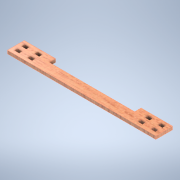
# Autodesk Inventor part: DoorFrameTop
Saved by Autodesk Inventor 2022.2 (Build 262287000, 287)
## iProperties
Created: 2023-03-05
Part Number: DoorFrameTop
Material: Wood (Oak)
Document SubType Name: Modeling
Designer: jaege
Density: 0.76 g/cm^3
Appearance: Red Oak - Natural Low Gloss
Author: jaege
Autodesk Inventor part; units mm, degrees
ref_plane "YZ Plane" through (0, 0, 0) normal (1, 0, 0) x (0, 1, 0)
ref_plane "XZ Plane" through (0, 0, 0) normal (0, 1, 0) x (-1, 0, 0)
ref_plane "XY Plane" through (0, 0, 0) normal (0, 0, 1) x (1, 0, 0)
sketch "Sketch1" plane through (0, 0, 0) normal (0, 1, 0) x (-1, 0, 0)
  line L0 (92, -20.8) -> (53, -20.8)
  line L1 (53, -20.8) -> (53, -12.8)
  line L2 (53, 0) -> (92, 0)
  line L3 (92, 0) -> (92, -20.8)
  line L4 (53, 0) -> (-53, 0)
  line L5 (-53, 0) -> (-53, -12.8) construction
  line L6 (-53, -12.8) -> (53, -12.8)
  line L7 (53, -12.8) -> (53, 0) construction
  line L8 (-53, 0) -> (-92, 0)
  line L9 (-92, 0) -> (-92, -20.8)
  line L10 (-92, -20.8) -> (-53, -20.8)
  line L11 (-53, -20.8) -> (-53, -12.8)
  line L12 (0, -12.8) -> (0, 0)
  line L13 (92, -16.8) -> (-92, -16.8) construction
  line L14 (92, -8) -> (-92, -8) construction
  line L15 (53, -12.8) -> (53, 0) construction
  line L16 (-53, -12.8) -> (-53, 0) construction
  line L17 (92, -4) -> (-92, -4) construction
  line L18 (87.5, -16.8) -> (81.5, -16.8)
  line L19 (81.5, -16.8) -> (81.5, -12.8)
  line L20 (81.5, -12.8) -> (87.5, -12.8)
  line L21 (87.5, -12.8) -> (87.5, -16.8)
  line L22 (71.5, -16.8) -> (65.5, -16.8)
  line L23 (65.5, -16.8) -> (65.5, -12.8)
  line L24 (65.5, -12.8) -> (71.5, -12.8)
  line L25 (71.5, -12.8) -> (71.5, -16.8)
  line L26 (-65.5, -16.8) -> (-71.5, -16.8)
  line L27 (-71.5, -16.8) -> (-71.5, -12.8)
  line L28 (-71.5, -12.8) -> (-65.5, -12.8)
  line L29 (-65.5, -12.8) -> (-65.5, -16.8)
  line L30 (-81.5, -16.8) -> (-87.5, -16.8)
  line L31 (-87.5, -16.8) -> (-87.5, -12.8)
  line L32 (-87.5, -12.8) -> (-81.5, -12.8)
  line L33 (-81.5, -12.8) -> (-81.5, -16.8)
  line L34 (87.5, -8) -> (81.5, -8)
  line L35 (81.5, -8) -> (81.5, -4)
  line L36 (81.5, -4) -> (87.5, -4)
  line L37 (87.5, -4) -> (87.5, -8)
  line L38 (71.5, -8) -> (65.5, -8)
  line L39 (65.5, -8) -> (65.5, -4)
  line L40 (65.5, -4) -> (71.5, -4)
  line L41 (71.5, -4) -> (71.5, -8)
  line L42 (-65.5, -8) -> (-71.5, -8)
  line L43 (-71.5, -8) -> (-71.5, -4)
  line L44 (-71.5, -4) -> (-65.5, -4)
  line L45 (-65.5, -4) -> (-65.5, -8)
  line L46 (-81.5, -8) -> (-87.5, -8)
  line L47 (-87.5, -8) -> (-87.5, -4)
  line L48 (-87.5, -4) -> (-81.5, -4)
  line L49 (-81.5, -4) -> (-81.5, -8)
  line L50 (92, -12.8) -> (-92, -12.8) construction
  dimension "d0" = 39
  dimension "d1" = 106
  dimension "d2" = 39
  dimension "d3" = 4
  dimension "d4" = 4
  dimension "d6" = 4.8
  dimension "d8" = 6
  dimension "d9" = 4.5
  dimension "d10" = 4.5
  dimension "d11" = 10
  dimension "d12" = 10
  dimension "d13" = 4
  dimension "d14" = 4
  constraints: 103 end point, 24 parallel, 21 point on line, 15 perpendicular, 12 horizontal, 10 vertical alignment, 3 collinear, 3 horizontal alignment, 2 midpoint
  measures "d0" distance of L0.start L0.end
  measures "d1" distance of L5.end L1.end
  measures "d2" distance of L9.end L10.end
  measures "d3" distance between parallel lines of L0 L13
  measures "d4" distance between parallel lines of L6 L13
  measures "d6" distance between parallel lines of L14 L6
  measures "d8" distance of L19.end L20.end
  measures "d9" distance from line of L3 L18.start
  measures "d10" horizontal distance of L9.end L30.end
  measures "d11" distance of L18.end L22.start
  measures "d12" distance of L30.start L26.end
  measures "d13" distance between parallel lines of L17 L14
  measures "d14" distance between parallel lines of L4 L17
extrude "Extrusion1" add sketch "Sketch1" along normal blind 4
body "Solid1"
